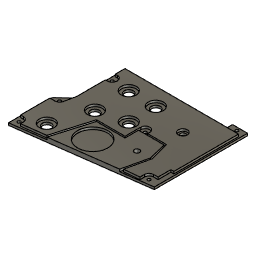
Panel - lower LG (Autodesk Fusion 360 design; units mm, degrees)
Autodesk Fusion 360 part; units mm, degrees
note: some values were not read from the file. Set by a fixed rule: which sketch regions a step uses.
sketch "Temp - LG panel" plane through (0, 0, 0) normal (0, 0, 1) x (1, 0, 0)
  line L0 (69, 67) -> (49, 67)
  line L1 (49, 59) -> (-86, 59)
  line L2 (-102, -22) -> (-102, -80)
  line L3 (69, -57) -> (69, 67)
  line L4 (49, 67) -> (49, 59)
  line L5 (-86, 59) -> (-86, -7)
  line L6 (-84, 44) -> (-81, 44)
  circle A0 centre (-24, -46) radius 18
  line L7 (-90, -76) -> (-59, -72)
  line L8 (-100, -27) -> (-100, -66)
  line L9 (30.4749, 19.5251) -> (43.6924, 6.3076)
  line L10 (-84, -7) -> (-87.0353, -22.1767)
  line L11 (28, 25.5) -> (28, 44.1924)
  line L12 (-3, 159) -> (-3, 69)
  line L13 (-14, 78) -> (-32, 78)
  line L14 (25.5251, 24.4749) -> (12.3076, 37.6924)
  line L15 (31.5, 22) -> (50.1924, 22)
  line L16 (51, -58) -> (51, -52)
  line L17 (63, -46) -> (63, -29)
  line L18 (-6, -21) -> (-6, 0)
  line L19 (67, 57) -> (-84, 57)
  line L20 (36, -29) -> (28.3503, -62.4675)
  line L21 (-71, 69) -> (-71, 140)
  line L22 (-32, 78) -> (-32, 116)
  line L23 (38, -29) -> (31, -60)
  line L24 (-71, 140) -> (-52, 159)
  line L25 (6, -3) -> (31, -3)
  line L26 (-75, 38) -> (-75, 37)
  line L27 (57, -46) -> (63, -46)
  arc A1 (51, -52) -> (57, -46) centre (57, -52) cw
  line L28 (-86, -7) -> (-102, -22)
  line L29 (-100, -66) -> (-96, -66)
  line L30 (-4, -23) -> (-4, -5)
  line L31 (-3, 69) -> (-71, 69)
  arc A2 (-11.0224, -56.981) -> (-36.9782, -56.9803) centre (-24.0007, -71.3763) ccw
  line L32 (30.4749, 24.4749) -> (43.6924, 37.6924)
  line L33 (-57, -74) -> (-42, -23)
  arc A3 (-38.4222, -37) -> (-9.5778, -37) centre (-24, -46) ccw
  line L34 (-84, 31) -> (-84, -7)
  arc A4 (-75, 37) -> (-81, 31) centre (-81, 37) cw
  line L35 (-4, -5) -> (30, -5)
  line L36 (-81, 31) -> (-84, 31)
  line L37 (-42, -23) -> (-4, -23)
  arc A5 (-96, -66) -> (-90, -72) centre (-96, -72) cw
  line L38 (-38.4222, -37) -> (-9.5778, -37)
  line L39 (-59, -72) -> (-44, -21)
  arc A6 (-16, -44) -> (-32, -44) centre (-24, -53.1667) ccw
  circle A7 centre (-24, -46) radius 20.0998
  line L40 (-52, 159) -> (-3, 159)
  line L41 (-84, 57) -> (-84, 44)
  line L42 (6, 0) -> (6, -3)
  line L43 (31, -3) -> (38, -29)
  line L44 (-32, 116) -> (-14, 116)
  line L45 (-102, -80) -> (69, -57)
  line L46 (-14, 116) -> (-14, 78)
  arc A8 (0, 6) -> (6, 0) centre (0, 0) cw
  line L47 (31, -60) -> (51, -58)
  arc A9 (-6, 0) -> (0, 6) centre (0, 0) cw
  line L48 (-44, -21) -> (-6, -21)
  line L49 (67, -29) -> (67, 57)
  line L50 (38, -29) -> (67, -29)
  line L51 (30, -5) -> (36, -29)
  line L52 (-90, -72) -> (-90, -76)
  line L53 (-92.9188, -27) -> (-100, -27)
  arc A10 (-81, 44) -> (-75, 38) centre (-81, 38) cw
  arc A11 (-87.0353, -22.1767) -> (-92.9188, -27) centre (-92.9188, -21) cw
  line L54 (35.0705, -57.014) -> (35.1868, -54.0004)
  arc A12 (36.9964, -41.3826) -> (35.0705, -57.014) centre (50.3943, -50.9677) ccw
  line L55 (35.0705, -57.014) -> (33.2225, -54.6307)
  line L56 (-13, 124) -> (-33, 124)
  line L57 (42, -23) -> (42, -7)
  line L58 (-62, 88) -> (-62, 106)
  line L59 (-33, 124) -> (-33, 146)
  line L60 (5.9161, 1) -> (67, 1)
  line L61 (-44, 88) -> (-62, 88)
  line L62 (-10, 149) -> (-10, 121)
  line L63 (-10, 121) -> (-36, 121)
  line L64 (-36, 121) -> (-36, 149)
  line L65 (-44, 106) -> (-44, 88)
  line L66 (42, -7) -> (60, -7)
  line L67 (-62, 106) -> (-44, 106)
  line L68 (60, -23) -> (42, -23)
  line L69 (-13, 146) -> (-13, 124)
  line L70 (-33, 146) -> (-13, 146)
  line L71 (60, -7) -> (60, -23)
  line L72 (-36, 149) -> (-10, 149)
  circle A13 centre (28, 22) radius 3.5
  circle A14 centre (-53, 97) radius 4
  circle A15 centre (28, 22) radius 16
  circle A16 centre (-23, 97) radius 6
  circle A17 centre (19, -30) radius 3.5
  line L73 (-32.5, 80) -> (-32.5, 114)
  circle A18 centre (-60, 135) radius 4
  circle A19 centre (-53, 97) radius 5.5
  circle A20 centre (-60, 135) radius 5.5
  circle A21 centre (-53, 97) radius 3
  line L74 (-27.0415, 90) -> (-31.0829, 97)
  line L75 (-13.5, 80) -> (-32.5, 80)
  line L76 (-27.0415, 104) -> (-25.5901, 104)
  line L77 (-22.9839, 96) -> (-23.0161, 96)
  line L78 (-32.5, 114) -> (-13.5, 114)
  arc A22 (-21.2995, 97.4703) -> (-22.9839, 96) centre (-22.9839, 97.7) cw
  line L79 (-63.5, -75) -> (-82.5, -75)
  line L80 (-20.4099, 104) -> (-18.9585, 104)
  line L81 (-18.9585, 104) -> (-14.9171, 97)
  circle A23 centre (-60, 135) radius 3
  circle A24 centre (-53, 97) radius 3
  circle A25 centre (-20, 34) radius 6
  circle A26 centre (-20, 34) radius 10
  circle A27 centre (-56, 34) radius 10
  circle A28 centre (-20.0161, -2) radius 10
  line L82 (-14.9171, 97) -> (-18.9585, 90)
  line L83 (-18.9585, 90) -> (-27.0415, 90)
  circle A29 centre (-73, -58) radius 6
  arc A30 (-23.0932, 107) -> (-20.4179, 103.9352) centre (-23.0932, 104.3) cw
  circle A31 centre (-23, 97) radius 8.5
  circle A32 centre (-20.0161, -2) radius 6
  circle A33 centre (-56, 34) radius 6
  circle A34 centre (-56, -11) radius 6
  line L84 (-13.5, 114) -> (-13.5, 80)
  circle A35 centre (-73, -58) radius 10
  line L85 (-24.7005, 97.4703) -> (-25.5821, 103.9352)
  circle A36 centre (-56, -11) radius 10
  line L86 (-20.4179, 103.9352) -> (-21.2995, 97.4703)
  arc A37 (-25.5821, 103.9352) -> (-22.9068, 107) centre (-22.9068, 104.3) cw
  line L87 (-31.0829, 97) -> (-27.0415, 104)
  line L88 (-22.9068, 107) -> (-23.0932, 107)
  arc A38 (-23.0161, 96) -> (-24.7005, 97.4703) centre (-23.0161, 97.7) cw
  circle A39 centre (19, -30) radius 6
  circle A40 centre (28, 22) radius 6
  circle A41 centre (-81, 37) radius 2
  circle A42 centre (-92.9188, -21) radius 2
  circle A43 centre (-96, -72) radius 2
  circle A44 centre (57, -52) radius 2
  circle A45 centre (0, 0) radius 2
  line L89 (49, 63) -> (69, 63) construction
  line L90 (59, 63) -> (59, 59.8803)
  circle A46 centre (59, 63) radius 2
  point P0 (1.7552, -0.1197)
  point P1 (1.7552, -0.1197)
  point P2 (1.7552, -0.1197)
  point P3 (1.7552, -0.1197)
  point P4 (1.7552, -0.1197)
  point P5 (1.7552, -0.1197)
  point P6 (1.7552, -0.1197)
  point P7 (1.7552, -0.1197)
  point P8 (1.7552, -0.1197)
  point P9 (1.7552, -0.1197)
  dimension "d1" = 20
  dimension "d8" = 12
  dimension "d9" = 7
  dimension "d10" = 12
  dimension "d17" = 4
  dimension "d21" = 4
  dimension "d26" = 20
  dimension "d28" = 69
  dimension "d29" = 155
  dimension "d30" = 2
  dimension "d31" = 87.7552
  constraint equal A26 A27
  constraint equal A27 A36
  constraint equal A27 A35
  constraint equal A27 A28
  constraint equal A25 A33
  constraint equal A32 A34
  constraint equal A33 A34
  constraint equal A29 A33
  constraint concentric A17 A39
  constraint equal A13 A17
  constraint concentric A15 A40
  constraint equal A39 A40
  constraint concentric A4 A41
  constraint concentric A11 A42
  constraint concentric A5 A43
  constraint concentric A1 A44
  constraint concentric A8 A45
  constraint equal A41 A45
  constraint equal A41 A44
  constraint equal A41 A42
  constraint equal A41 A43
  constraint midpoint L4 L89.start
  constraint perpendicular L3 L89
  constraint horizontal L89
  constraint coincident L3 L89.end
  constraint midpoint L89 L90.start
  constraint perpendicular L89 L90
  constraint coincident L90.start A46.centre
  constraint equal A45 A46
  measures "d1" diameter of A27
  measures "d8" diameter of A39
  measures "d9" diameter of A17
  measures "d10" diameter of A33
  measures "d17" diameter of A41
  measures "d21" distance of L0 L89
  measures "d26" distance of L3 L4
  measures "d28" distance of L3 A8.centre
  measures "d29" distance of L3 L5
  measures "d30" distance of L3 L49
  measures "d31" distance of L5 P9
extrude "Extrude1" add sketch "Temp - LG panel" along normal blind 6 contours L20 L30 L33 L35 L37 L45 L51 | L6 L7 L8 L10 L18 L19 L26 L29 L34 A4 L36 A5 L39 L41 A8 A9 L48 L49 L52 L53 A10 A11 L60 | L25 L42 L43 A8 L49 L50 L60 | L16 L17 L23 L27 A1 L47 L50 | A39 makes body 1 at (57, 24, 0) makes body 2 at (14.1489, -48.2918, 0)
extrude "Extrude2" add sketch "Temp - LG panel" along normal blind 3 contours L0 L1 L2 L3 L4 L5 L20 L28 L30 L33 L35 L37 L45 L51 | A41 | A42 | A43 | A44 | A45 | A46 bodies 1 2
extrude "Extrude3" add sketch "Temp - LG panel" along normal blind 3 contours A26 | A27 | A28 | A35 | A36 bodies 1
extrude "Extrude4" add sketch "Temp - LG panel" along normal blind 6 contours L9 L15 A15 A40 | L9 L14 A15 A40 | L11 L14 A15 A40 | L15 L32 A15 A40 | L11 L32 A15 A40 bodies 1
extrude "Extrude5" add sketch "Temp - LG panel" along normal blind 3 contours L9 L15 A13 A40 | L9 L14 A13 A40 | L11 L14 A13 A40 | L15 L32 A13 A40 | L11 L32 A13 A40 bodies 1
extrude "Extrude6" add sketch "Temp - LG panel" along normal blind 6 contours L57 L66 L68 L71 bodies 1
extrude "Extrude7" cut sketch "Temp - LG panel" along normal through all contours A41 | A42 | A43 | A44 | A45 bodies 1
extrude "Extrude8" add sketch "Temp - LG panel" along normal blind 3 contours A0 | A2 A3 | A2 A3 L38 | A7 bodies 1
extrude "Extrude9" cut sketch "Temp - LG panel" along normal through all contours A46 bodies 1
named bodies: "Panel - lower LG"
